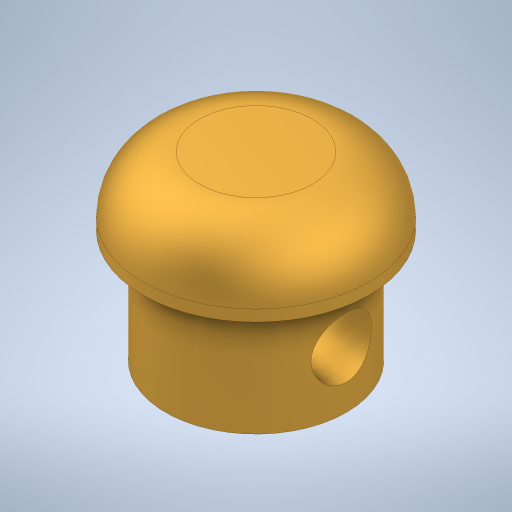
# Autodesk Inventor part: Brass Endweight
Saved by Autodesk Inventor 2023 (Build 270158000, 158)
## iProperties
Created: 2023-02-13
Part Number: Brass Endweight
Material: Brass, Soft Yellow
Document SubType Name: Modeling
Designer: mbear
Density: 8.47 g/cm^3
Appearance: Brass - Satin
Mass: 7.79901 g
Surface Area: 5.49195 cm^2
Volume: 0.920781 cm^3
Author: mbear
Autodesk Inventor part; units mm, degrees
ref_plane "XZ Plane" through (0, 0, 0) normal (0, 1, 0) x (-1, 0, 0)
ref_plane "XY Plane" through (0, 0, 0) normal (0, 0, 1) x (1, 0, 0)
sketch "Sketch1" plane through (0, 0, 0) normal (0, 1, 0) x (-1, 0, 0)
  circle A0 centre (0, 0) radius 5.08
  dimension "d0" = 10.16
  constraints: 1 centre point, 1 coincident
  measures "d0" diameter of A0
extrude "Extrusion1" add sketch "Sketch1" along normal blind 6.35
sketch "Sketch2" plane through (0, 6.35, 0) normal (0, 1, 0) x (1, 0, 0)
  circle A0 centre (0, 0) radius 6.35
  dimension "d3" = 12.7
  constraints: 1 centre point, 1 coincident
  measures "d3" diameter of A0
extrude "Extrusion2" add sketch "Sketch2" along normal blind 3.81
fillet "Fillet1" radius 3.175 1 edges at (-6.35, 10.16, 0)
ref_plane "Work Plane1" through (5.08, 0, 0) normal (1, 0, 0) x (0, 1, 0)
sketch "Sketch3" plane through (5.08, 0, 0) normal (1, 0, 0) x (0, 1, 0)
  circle A0 centre (3.175, 0) radius 0.726
  point P0 (0, 0)
  dimension "d8" = 3.175
  constraints: 1 centre point
  measures "d8" distance of A0.centre point (0, 0)
hole "Hole1" at (5.08, 3.175, 0) direction (-1, 0, 0) diameter 3.4 depth 25.4 tip angle 118 clearance for "Socket Head Cap Screw" size "M3" standard "Ansi Metric M Profile"
body "Solid1"
